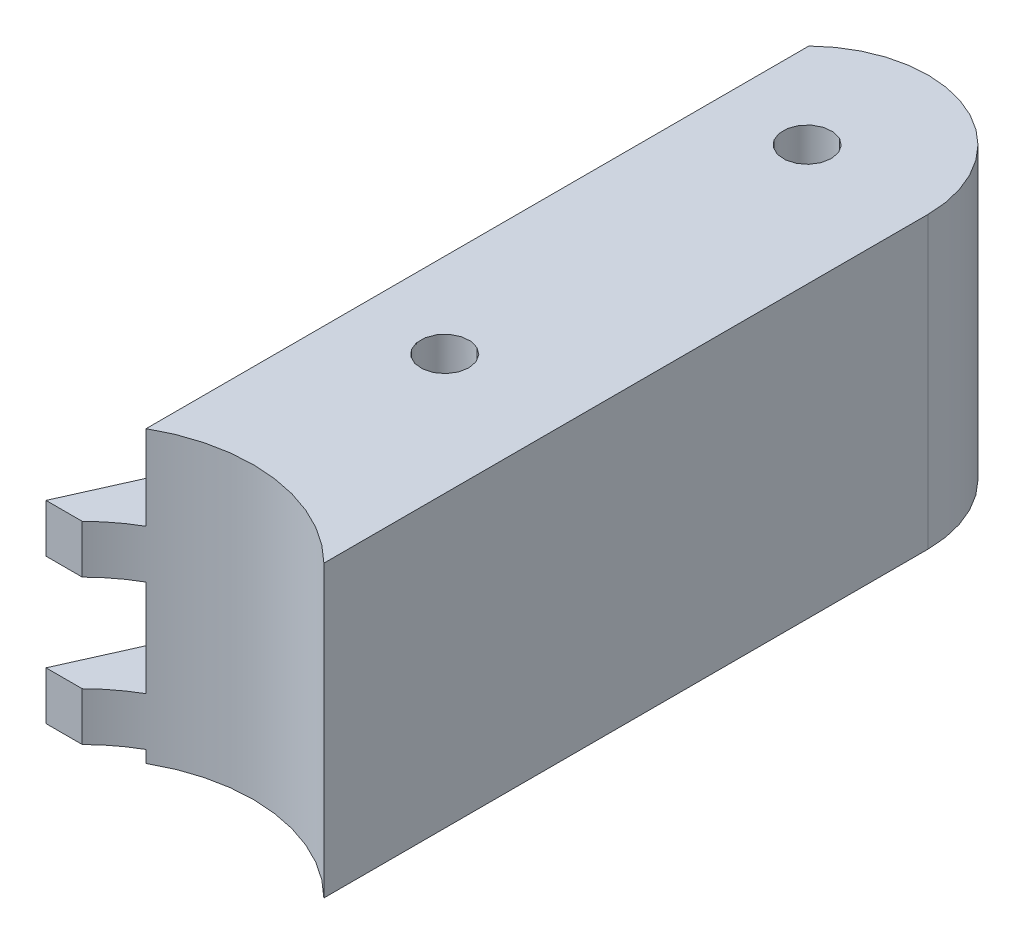
# Autodesk Inventor part: clawGrip
Saved by Autodesk Inventor 2023 (Build 270158030, 158C)
## iProperties
Created: 2023-03-03
Part Number: clawGrip
Material: Rubber
Document SubType Name: Modeling
Designer: kumpu
Density: 0.93 g/cm^3
Appearance: Rubber - Black
Author: kumpu
Autodesk Inventor part; units mm, degrees
ref_plane "YZ Plane" through (0, 0, 0) normal (1, 0, 0) x (0, 1, 0)
ref_plane "XZ Plane" through (0, 0, 0) normal (0, 1, 0) x (-1, 0, 0)
ref_plane "XY Plane" through (0, 0, 0) normal (0, 0, 1) x (1, 0, 0)
sketch "Sketch1" plane through (0, 0, 0) normal (0, 0, 1) x (1, 0, 0)
  line L0 (-17, 0) -> (-17, 1)
  line L1 (-17, 1) -> (-23, 1)
  line L2 (-23, 1) -> (-23, 5)
  line L3 (-23, 5) -> (-17, 5)
  line L4 (-17, 5) -> (-17, 13)
  line L5 (-17, 13) -> (-23, 13)
  line L6 (-23, 13) -> (-23, 17)
  line L7 (-23, 17) -> (-17, 17)
  line L8 (-17, 17) -> (-17, 24)
  line L9 (-17, 24) -> (0, 24)
  line L10 (0, 24) -> (0, 0)
  line L11 (0, 0) -> (-17, 0)
  dimension "d0" = 4
  dimension "d1" = 17
  dimension "d2" = 1
  dimension "d3" = 24
  dimension "d4" = 6
  dimension "d5" = 8
  constraints: 24 end point, 8 perpendicular, 6 point on line, 1 coincident, 1 collinear, 1 vertical
  measures "d0" distance of L1.end L2.end
  measures "d1" distance of L10.end L0.start
  measures "d2" distance of L0.start L0.end
  measures "d3" distance of L9.end L10.end
  measures "d4" distance of L6.end L7.end
  measures "d5" distance of L3.end L4.end
extrude "Extrusion1" add sketch "Sketch1" along normal blind 50
sketch "Sketch2" plane through (-17, 24, 0) normal (0, 1, 0) x (1, 0, 0)
  line L0 (17, 0) -> (0, 0) projected
  line L1 (0, 0) -> (0, -50) projected
  line L2 (0, 0) -> (17, 0) projected
  line L3 (0, 0) -> (0, 7.1414)
  line L4 (17, 0) -> (17, -50) projected
  line L5 (0, 0) -> (17, 0)
  arc A0 (17, 0) -> (0, 7.1414) centre (7, 0) ccw
  dimension "d9" = 10
  constraints: 4 end point, 2 point on circle, 1 centre point, 1 horizontal, 1 tangent, 1 vertical
  measures "d9" radius of A0
extrude "Extrusion2" add sketch "Sketch2" against normal blind 24
sketch "Sketch3" plane through (-17, 24, 50) normal (0, 1, 0) x (1, 0, 0)
  arc A0 (17, 50) -> (0, 57.1414) centre (7, 50) ccw projected
  circle A1 centre (7, 50) radius 2
  circle A2 centre (7, 20) radius 2
  line L0 (0, 50) -> (0, 0) projected
  line L1 (7, 50) -> (7, -10) construction
  line L2 (17, 0) -> (0, 0) construction
  arc A3 (17, 0) -> (-3, 0) centre (7, -10) ccw
  line L3 (17, 50) -> (17, 0) construction
  line L4 (-3, 0) -> (17, 0)
  line L5 (-6, 50) -> (-6, 0) construction
  line L6 (-6, 11.4006) -> (-6, 28.5994)
  arc A4 (-6, 11.4006) -> (-6, 28.5994) centre (-29.9, 20) ccw
  line L7 (7, 20) -> (-4.5, 20) construction
  line L8 (-6, 0) -> (-3.4507, 5.7003)
  line L9 (-3.4507, 5.7003) -> (-6, 11.4006)
  line L10 (-6, 28.5994) -> (-3.7582, 33.612)
  line L11 (-3.7582, 33.612) -> (-6, 38.6246)
  line L12 (-6, 38.6246) -> (-3.4563, 44.3123)
  line L13 (-3.4563, 44.3123) -> (-6, 50)
  line L14 (-6, 0) -> (-6, 11.4006)
  line L15 (-6, 28.5994) -> (-6, 38.6246)
  line L16 (-6, 38.6246) -> (-6, 50)
  dimension "d12" = 4
  dimension "d13" = 60
  dimension "d14" = 11.5
  dimension "d15" = 25.4
  constraints: 26 end point, 5 point on circle, 4 centre point, 4 collinear, 3 coincident, 3 equal length, 2 horizontal, 2 parallel, 2 point on line, 2 vertical, 1 equal radius, 1 midpoint
  measures "d12" diameter of A1
  measures "d13" distance of L1.start L1.end
  measures "d14" distance of L7.start L7.end
  measures "d15" radius of A4
extrude "Extrusion3" cut sketch "Sketch3" against normal through all
body "Solid1"
